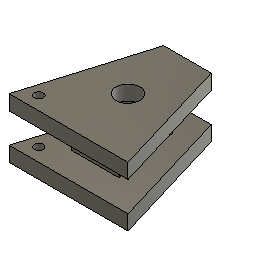
Bobin Birleşik v5 (Autodesk Fusion 360 design; units mm, degrees)
Autodesk Fusion 360 part; units mm, degrees
sketch "Eskiz1" plane through (0, 0, 0) normal (0, 1, 0) x (1, 0, 0)
  line L0 (0, 0) -> (40, 0)
  line L1 (40, 0) -> (40, -40)
  line L2 (40, -40) -> (0, -40)
  line L3 (0, -40) -> (0, 0)
  line L4 (12, 0) -> (35, 0)
  line L5 (35, -40) -> (12, -40)
  line L6 (12, -40) -> (12, 0)
  line L7 (28, 0) -> (28, -40)
  line L8 (12, 0) -> (0, -40)
  line L9 (28, 0) -> (40, -40)
  circle A0 centre (20, -20) radius 4
  point P0 (12, 0)
  point P1 (28, 0)
  dimension "d1" = 40
  dimension "d2" = 40
  dimension "d3" = 12
  dimension "d4" = 12
  dimension "d5" = 40
  dimension "d23" = 8
  constraint horizontal L0
  constraint vertical L1
  constraint horizontal L2
  constraint vertical L3
  constraint coincident L0.start L3.end
  constraint coincident L0 P0
  constraint coincident L0 P1
  constraint horizontal L4
  constraint horizontal L5
  constraint vertical L6
  constraint coincident L2 L5.start
  constraint coincident P0 L4.start
  constraint vertical L7
  constraint coincident P1 L7.start
  measures "d1" distance of L0.start L0.end
  measures "d2" distance of L0.start L2.end
  measures "d3" distance of L0.start L4.start
  measures "d4" distance of L0.end P1
  measures "d5" distance of P1 L7.end
  measures "d23" diameter of A0
extrude "Ekstrüde Et1" add sketch "Eskiz1" along normal blind 5 contours L0 L2 L4 L5 L6 L7 | L2 L6 L8 | L2 L5 L7 L9 | A0 makes body 1
sketch "Eskiz2" plane through (0, 5, 0) normal (0, 1, 0) x (-1, 0, 0)
  line L0 (-12, 0) -> (0, 40)
  line L1 (0, 40) -> (-40, 40)
  line L2 (-40, 40) -> (-28, 0)
  line L3 (-28, 0) -> (-12, 0)
  line L4 (-12, 0) -> (-28, 0)
  line L5 (-28, 0) -> (-28, 40)
  line L6 (-28, 40) -> (-12, 40)
  line L7 (-12, 40) -> (-12, 0)
  line L8 (-12, 31) -> (-28, 31)
  line L9 (-16, 9) -> (-12, 31)
  line L10 (-24, 9) -> (-28, 31)
  line L11 (-16, 9) -> (-24, 9)
  circle A0 centre (-5.5, 35.5) radius 1.5
  point P0 (-16, 9)
  point P1 (-24, 9)
  point P2 (-12, 35.5)
  point P3 (-5.5, 35.5)
  dimension "d8" = 16
  dimension "d9" = 40
  dimension "d16" = 4
  dimension "d17" = 4
  dimension "d18" = 9
  dimension "d19" = 9
  dimension "d20" = 9
  dimension "d33" = 6.5
  dimension "d34" = 4.5
  dimension "d35" = 3
  constraint horizontal L4
  constraint vertical L5
  constraint horizontal L6
  constraint vertical L7
  constraint coincident L0.start L3.end
  constraint coincident L7 L8.start
  constraint coincident L5 L8.end
  constraint perpendicular L5 L8
  constraint coincident P0 L9.start
  constraint coincident P1 L10.start
  constraint coincident L7 P2
  constraint coincident P3 A0.centre
  measures "d8" distance of L0.start L2.end
  measures "d9" distance of L0.start L6.end
  measures "d16" distance of L7 P0
  measures "d17" distance of L5 P1
  measures "d18" distance of L4 P1
  measures "d19" distance of L4 P0
  measures "d20" distance of L6 L8
  measures "d33" distance of P2 P3
  measures "d34" distance of L8 P2
  measures "d35" diameter of A0
copy_body "CopyPasteBodies1" bodies 1 makes body 2
extrude "Ekstrüde Et4" add sketch "Eskiz2" along normal blind 10 contours L8 L9 L10 L11 bodies 1
move_body "Taşı1" bodies 2 to x (1, 0, 0) y (0, 1, 0) z (0, 0, 1) at (0, 15, 0)
extrude "Ekstrüde Et5" cut sketch "Eskiz1" along normal blind 25 contours A0 bodies 1 2
extrude "Ekstrüde Et6" cut sketch "Eskiz2" along normal blind 19 and the other way blind 8.5 contours A0 bodies 1 2
